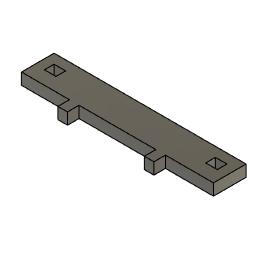
North + South Plank v1 (Autodesk Fusion 360 design; units mm, degrees)
Autodesk Fusion 360 part; units mm, degrees
sketch "Sketch1" plane through (0, 0, 0) normal (0, 0, 1) x (1, 0, 0)
  line L0 (-45, 8.5) -> (45, 8.5)
  line L1 (45, 8.5) -> (45, -8.5)
  line L2 (45, -8.5) -> (-45, -8.5)
  line L3 (-45, -8.5) -> (-45, 8.5)
  line L4 (-45, 8.5) -> (45, -8.5) construction
  line L5 (45, 8.5) -> (-45, -8.5) construction
  dimension "d1" = 90
  dimension "d2" = 17
  constraint horizontal L0
  constraint perpendicular L0 L1
  constraint parallel L0 L2
  constraint parallel L1 L3
  constraint coincident L4 origin
  constraint coincident L5 origin
  measures "d1" distance of L1.end L2.end
  measures "d2" distance of L0.end L1.end
extrude "Extrude1" add sketch "Sketch1" along normal blind 6
sketch "Sketch2" plane through (0, 0, 6) normal (0, 0, 1) x (-1, 0, 0)
  line L0 (45, 8.5) -> (-45, 8.5)
  line L1 (-45, 8.5) -> (-45, -8.5)
  line L2 (-45, -8.5) -> (45, -8.5)
  line L3 (45, -8.5) -> (45, 8.5)
  line L4 (45, -8.5) -> (39, -8.5) construction
  line L5 (39, -8.5) -> (39, -3.5) construction
  line L6 (39, -3.5) -> (45, -3.5) construction
  line L7 (45, -3.5) -> (45, -8.5) construction
  line L8 (-45, -8.5) -> (-39, -8.5) construction
  line L9 (-39, -8.5) -> (-39, -3.5) construction
  line L10 (-39, -3.5) -> (-45, -3.5) construction
  line L11 (-45, -3.5) -> (-45, -8.5) construction
  line L12 (45, -3.5) -> (39, -3.5)
  line L13 (39, -3.5) -> (39, 1.5)
  line L14 (39, 1.5) -> (45, 1.5)
  line L15 (45, 1.5) -> (45, -3.5)
  line L16 (-45, -3.5) -> (-39, -3.5)
  line L17 (-39, -3.5) -> (-39, 1.5)
  line L18 (-39, 1.5) -> (-45, 1.5)
  line L19 (-45, 1.5) -> (-45, -3.5)
  dimension "d5" = 6
  dimension "d6" = 5
  dimension "d7" = 6
  dimension "d8" = 5
  dimension "d9" = 5
  dimension "d10" = 5
  constraint horizontal L4
  constraint vertical L5
  constraint horizontal L6
  constraint vertical L7
  constraint coincident L2.end L3.start
  constraint horizontal L8
  constraint vertical L9
  constraint horizontal L10
  constraint vertical L11
  constraint coincident L1.end L2.start
  constraint horizontal L12
  constraint vertical L13
  constraint horizontal L14
  constraint vertical L15
  constraint horizontal L16
  constraint vertical L17
  constraint horizontal L18
  constraint vertical L19
  measures "d5" distance of L2.end L4.end
  measures "d6" distance of L2.end L6.end
  measures "d7" distance of L1.end L8.end
  measures "d8" distance of L1.end L10.end
  measures "d9" distance of L6.end L14.end
  measures "d10" distance of L10.end L18.end
extrude "Extrude2" cut sketch "Sketch2" against normal blind 9 contours L3 L12 L13 L14 L15 | L1 L16 L17 L18 L19
sketch "Sketch3" plane through (0, -8.5, 0) normal (0, -1, 0) x (1, 0, 0)
  line L0 (-45, 0) -> (45, 0)
  line L1 (45, 0) -> (45, 6)
  line L2 (45, 6) -> (-45, 6)
  line L3 (-45, 6) -> (-45, 0)
  line L4 (0, 6) -> (39, 6) construction
  line L5 (39, 0) -> (39, 6) construction
  line L6 (0, 6) -> (-39, 6) construction
  line L7 (-39, 6) -> (-39, 0) construction
  line L8 (0, 6) -> (0, 0)
  line L9 (0, 2.5249) -> (-20, 2.5249) construction
  line L10 (-20, 2.5249) -> (-20, 0) construction
  line L11 (0, 2.5249) -> (20, 2.5249) construction
  line L12 (-20, 0) -> (-25, 0)
  line L13 (-25, 0) -> (-25, 6)
  line L14 (-25, 6) -> (-20, 6)
  line L15 (-20, 6) -> (-20, 0)
  line L16 (20, 0) -> (25, 0)
  line L17 (25, 0) -> (25, 6)
  line L18 (25, 6) -> (20, 6)
  line L19 (20, 6) -> (20, 0)
  constraint midpoint L2 L4.start
  constraint coincident L2 L4.end
  constraint parallel L2 L4
  constraint coincident L0 L5.start
  constraint perpendicular L4 L5
  constraint coincident L2 L6.end
  constraint perpendicular L5 L6
  constraint coincident L0 L7.end
  constraint perpendicular L0 L7
  constraint coincident L8.end origin
  constraint coincident L8 L9.start
  constraint perpendicular L8 L9
  constraint coincident L0 L10.end
  constraint perpendicular L0 L10
  constraint perpendicular L8 L11
  constraint horizontal L12
  constraint vertical L13
  constraint horizontal L14
  constraint vertical L15
  constraint coincident L6 L13.end
  constraint horizontal L16
  constraint vertical L17
  constraint horizontal L18
  constraint vertical L19
  constraint coincident L4 L17.end
  constraint coincident L0 L16.start
extrude "Extrude3" add sketch "Sketch3" along normal blind 6 contours L0 L2 L12 L13 L14 L15 | L0 L2 L16 L17 L18 L19
sketch "Sketch4" plane through (-45, 0, 0) normal (-1, 0, 0) x (0, -1, 0)
  line L0 (-3.5, 0) -> (-3.5, 6)
  line L1 (-3.5, 6) -> (-8.5, 6)
  line L2 (-8.5, 6) -> (-8.5, 0)
  line L3 (-8.5, 0) -> (-3.5, 0)
  line L4 (-8.5, 6) -> (8.5, 6)
  line L5 (8.5, 6) -> (8.5, 0)
  line L6 (8.5, 0) -> (-8.5, 0)
  line L7 (-8.5, 0) -> (-8.5, 6)
  dimension "d15" = 17
  dimension "d16" = 6
  constraint horizontal L4
  constraint vertical L5
  constraint horizontal L6
  constraint vertical L7
  constraint coincident L1.end L2.start
  measures "d15" distance of L1.end L4.end
  measures "d16" distance of L1.end L2.end
extrude "Extrude4" add sketch "Sketch4" along normal blind 5
sketch "Sketch5" plane through (45, 0, 0) normal (1, 0, 0) x (0, 1, 0)
  line L0 (-1.5, 0) -> (-1.5, 6)
  line L1 (-1.5, 6) -> (-8.5, 6)
  line L2 (-8.5, 6) -> (-8.5, 0)
  line L3 (-8.5, 0) -> (-1.5, 0)
  line L4 (-8.5, 6) -> (8.5, 6)
  line L5 (8.5, 6) -> (8.5, 0)
  line L6 (8.5, 0) -> (-8.5, 0)
  line L7 (-8.5, 0) -> (-8.5, 6)
  dimension "d19" = 17
  constraint horizontal L4
  constraint vertical L5
  constraint horizontal L6
  constraint vertical L7
  constraint coincident L1.end L2.start
  measures "d19" distance of L1.end L4.end
extrude "Extrude5" add sketch "Sketch5" along normal blind 5
